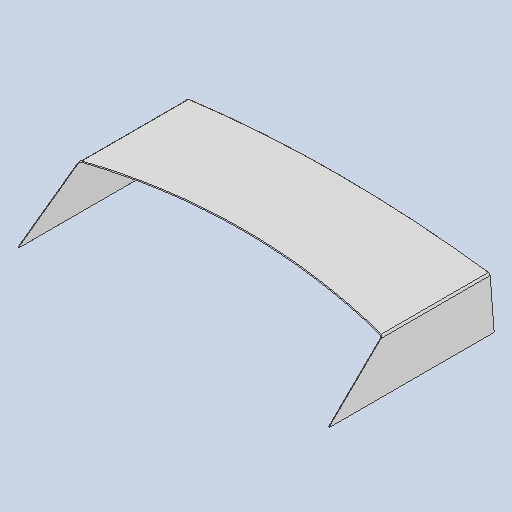
# Autodesk Inventor part: MSC 202 BACK-NECK
Saved by Autodesk Inventor 2025 (Build 290162010, 162A)
## iProperties
Created: 2024-04-18
Part Number: MSC 202 BACK-NECK
Material: Stainless Steel AISI 304
Document SubType Name: Sheet Metal
Designer: admin
Stock Number: МОО 202 СПИНА лист холка
Density: 8 g/cm^3
Flat Pattern Width: 198.003 cm
Flat Pattern Length: 81.5523 cm
Flat Pattern Area: 16147.6 cm^2
Sheet Metal Rule: Default_mm
Sheet Metal Width: 1980,030 mm
Sheet Metal Length: 815,523 mm
Sheet Metal Area: 1614761,012 mm^2
Appearance: Default
Mass: 25524.2 g
Surface Area: 21470.8 cm^2
Volume: 3190.53 cm^3
Author: admin
Autodesk Inventor part; units mm, degrees
ref_plane "YZ Plane" through (0, 0, 0) normal (1, 0, 0) x (0, 1, 0)
ref_plane "XZ Plane" through (0, 0, 0) normal (0, 1, 0) x (-1, 0, 0)
ref_plane "XY Plane" through (0, 0, 0) normal (0, 0, 1) x (1, 0, 0)
sketch "Sketch1" plane through (0, 0, 0) normal (0, 0, 1) x (1, 0, 0)
  line L0 (-750, 241.9) -> (750, 241.9) construction
  line L1 (750, 241.9) -> (750, -2458.1) construction
  line L2 (750, -2458.1) -> (-750, -2458.1) construction
  line L3 (-750, -2458.1) -> (-750, 241.9) construction
  line L4 (800, 291.9) -> (-800, 291.9) construction
  line L5 (-800, 291.9) -> (-800, -2508.1) construction
  line L6 (-800, -2508.1) -> (800, -2508.1) construction
  line L7 (800, -2508.1) -> (800, 291.9) construction
  line L8 (-850, 341.9) -> (850, 341.9) construction
  line L9 (850, 341.9) -> (850, -2558.1) construction
  line L10 (850, -2558.1) -> (-850, -2558.1) construction
  line L11 (-850, -2558.1) -> (-850, 341.9) construction
  arc A0 (750, 241.9) -> (742.111681, 242.950817) centre (0, -5358.1) ccw construction
  line L12 (-750, -1858.1) -> (750, -1858.1) construction
  line L13 (115.485997, -2455.9227) -> (750, -1858.1) construction
  arc A1 (750, -1858.1) -> (750, 241.9) centre (-10250, -808.1) ccw construction
  arc A2 (110, -2458.1) -> (115.485997, -2455.9227) centre (110, -2450.1) ccw construction
  arc A3 (742.111681, 242.950817) -> (0, 291.9) centre (0, -5358.1) ccw
  line L14 (0, 341.9) -> (0, 291.9) construction
  line L15 (0, -2458.1) -> (0, -2455.1) construction
  line L16 (0, 288.9) -> (0, 241.9) construction
  line L17 (0, 291.9) -> (0, 288.9) construction
  line L18 (750.763103, 233.874638) -> (770.411716, 0)
  arc A4 (750.763103, 233.874638) -> (742.111681, 242.950817) centre (740.798209, 233.037453) ccw
  point P0 (0, 0)
  point P1 (0, -2508.1)
  dimension "d134" = 1500
  dimension "d135" = 2700
  dimension "d136" = 2100
  dimension "d137" = 8
  dimension "d138" = 50
  dimension "d139" = 50
  dimension "d140" = 3
  dimension "d141" = 10
  dimension "d142" = 241.9
  measures "d134" distance of L3.end L1.start
  measures "d135" distance of L1.start L2.start
  measures "d136" distance between parallel lines of L12 L0
  measures "d137" radius of A2
  measures "d138" distance between parallel lines of L4 L8
  measures "d139" distance between parallel lines of L0 L4
  measures "d140" distance of L17.start L16.start
  measures "d141" radius of A4
  measures "d142" vertical distance of L18.end L1.start
contour flange "Contour Flange2" sketch "Sketch1" thickness 3 bend radius 3 width 819 along (0, 0, 1) mid plane no both sides no wall seen from (760.58741, 116.937319, 0) lies toward (-0.9964894, -0.0837185, 0) curves L18 A4 A3
bend "Bend2"
corner "Corner2"
mirror "Mirror2" about plane through (0, 0, 0) normal (1, 0, 0) of "Contour Flange2"
sketch "Sketch2" plane through (0, 0, 0) normal (1, 0, 0) x (0, 1, 0)
  line L0 (499.748844, 819) -> (-0.251156, 819)
  line L1 (499.748844, 223.123204) -> (499.748844, 819)
  line L2 (499.748844, 223.123204) -> (-0.251156, 819)
  line L3 (-0.251156, 819) -> (-0.251156, 0)
  point P0 (0, 0)
  dimension "d149" = 40
  dimension "d150" = 500
  constraints: 6 end point, 2 perpendicular
  measures "d149" angle of L3 L2
  measures "d150" distance between parallel lines of L3 L1
extrude "Extrusion2" cut sketch "Sketch2" along normal through all both and the other way through all
fillet "Fillet1" radius 2 2 edges at (-768.917, -0.1256, 818.8503) (768.917, -0.1256, 818.8503)
sketch "Sketch4" plane through (-747.773635, 233.623482, 540.27906) normal (0.9964894, -0.0837185, 0) x (0, 0, -1)
  line L0 (-273.234352, -234.69856) -> (540.27906, -234.69856)
  line L1 (540.27906, -234.69856) -> (540.27906, 0)
  line L2 (416.776539, -231.867046) -> (360.277479, -231.867046) construction
  line L3 (360.277479, -231.867046) -> (360.277479, -227.342447) construction
  line L4 (360.277479, -227.342447) -> (416.776539, -227.342447) construction
  line L5 (416.776539, -227.342447) -> (416.776539, -231.867046) construction
  point P0 (540.27906, -170.200843)
  constraints: 2 other
mark "Mark2"
equation "\"d36\" = Thickness"
equation "\"d37\" = BendReliefWidth"
equation "\"d38\" = BendReliefDepth"
equation "\"d39\" = MinimumRemnant"
equation "\"d40\" = TransitionRadius"
equation "\"d42\" = BendRadius"
equation "\"d44\" = CornerReliefSize"
equation "\"d45\" = GapSize"
equation "\"d46\" = JacobiRadiusSize"
equation "\"BendRadius\" = Thickness"
equation "\"BendReliefWidth\" = Thickness"
equation "\"BendReliefDepth\" = 0.5 * Thickness"
equation "\"CornerReliefSize\" = 4 * Thickness"
equation "\"MinimumRemnant\" = 2 * Thickness"
equation "\"TransitionRadius\" = BendRadius"
equation "\"JacobiRadiusSize\" = BendRadius"
equation "\"GapSize\" = Thickness"
equation "\"Thickness\" = 3"
body "Solid3"
